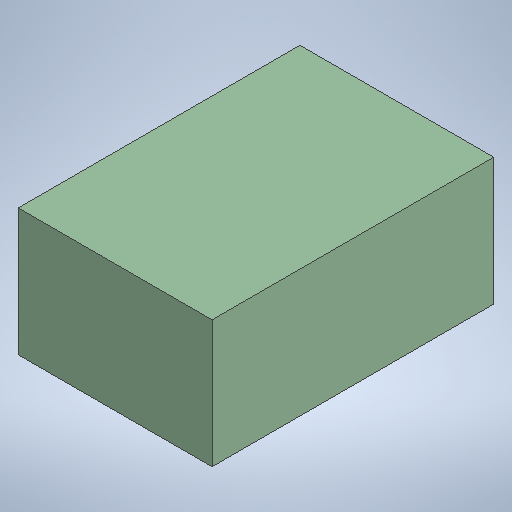
# Autodesk Inventor part: RasPi
Saved by Autodesk Inventor 2025.1 (Build 291241000, 241)
## iProperties
Created: 2025-02-21
Part Number: RasPi
Material: Generic
Document SubType Name: Modeling
Designer: m_kni
Density: 1 g/cm^3
Appearance: Default
Author: m_kni
Autodesk Inventor part; units mm, degrees
ref_plane "YZ Plane" through (0, 0, 0) normal (1, 0, 0) x (0, 1, 0)
ref_plane "XZ Plane" through (0, 0, 0) normal (0, 1, 0) x (-1, 0, 0)
ref_plane "XY Plane" through (0, 0, 0) normal (0, 0, 1) x (1, 0, 0)
sketch "Sketch1" plane through (0, 0, 0) normal (0, 1, 0) x (-1, 0, 0)
  line L0 (-32, -46.5) -> (32, -46.5)
  line L1 (32, -46.5) -> (32, 46.5)
  line L2 (32, 46.5) -> (-32, 46.5)
  line L3 (-32, 46.5) -> (-32, -46.5)
  line L4 (-32, -46.5) -> (32, 46.5) construction
  line L5 (32, -46.5) -> (-32, 46.5) construction
  point P0 (0, 0)
  dimension "d0" = 64
  dimension "d1" = 93
  constraints: 12 end point, 2 midpoint, 2 parallel, 1 horizontal, 1 perpendicular
  measures "d0" distance of L2.end L1.end
  measures "d1" distance of L1.end L0.end
extrude "Extrusion1" add sketch "Sketch1" along normal blind 42
body "Solid1"
